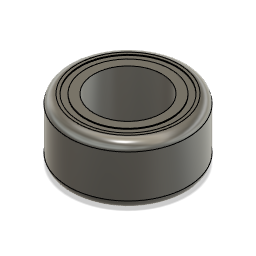
dualTriggerRemote v15 (Autodesk Fusion 360 archive; units mm, degrees)
design "smallBearing"
Autodesk Fusion 360 part; units mm, degrees
sketch "Sketch1" plane through (0, 0, 0) normal (0, 1, 0) x (1, 0, 0)
  circle A0 centre (0, 0) radius 7
  circle A1 centre (0, 0) radius 4
  dimension "d1" = 14
  dimension "d2" = 8
  constraint coincident A0.centre A1.centre
  measures "d1" diameter of A0
  measures "d2" diameter of A1
extrude "Extrude1" add sketch "Sketch1" along normal blind 7
fillet "Fillet1" radius 1 2 edges at (-6.5263, 0, 2.5313) (-6.5263, 7, 2.5313)
sketch "Sketch2" plane through (0, 7, 0) normal (0, 1, 0) x (-1, 0, 0)
  circle A0 centre (0, 0) radius 4
  circle A1 centre (0, 0) radius 6
  circle A2 centre (0, 0) radius 5.6638
  circle A3 centre (0, 0) radius 5
  constraint concentric A0 A2
  constraint concentric A0 A3
extrude "Extrude2" cut sketch "Sketch2" against normal blind 0.1 contours A2
sketch "Sketch3" plane through (0, 0, 0) normal (0, -1, 0) x (1, 0, 0)
  circle A0 centre (0, 0) radius 4
  circle A1 centre (0, 0) radius 6
  circle A2 centre (0, 0) radius 5
  circle A3 centre (0, 0) radius 5.6638
extrude "Extrude3" cut sketch "Sketch3" against normal blind 0.2 contours A3

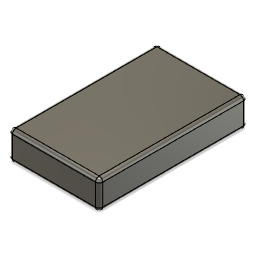
design "battery"
Autodesk Fusion 360 part; units mm, degrees
sketch "Sketch1" plane through (0, 0, 0) normal (0, 1, 0) x (1, 0, 0)
  line L0 (0, 0) -> (25, 0)
  line L1 (25, 0) -> (25, 41)
  line L2 (25, 41) -> (0, 41)
  line L3 (0, 41) -> (0, 0)
  dimension "d1" = 25
  dimension "d2" = 41
  constraint horizontal L0
  constraint vertical L1
  constraint horizontal L2
  constraint vertical L3
  constraint coincident L0.start L3.end
  measures "d1" distance of L0.start L0.end
  measures "d2" distance of L0.start L2.end
extrude "Extrude1" add sketch "Sketch1" along normal blind 8
fillet "Fillet1" radius 1 12 edges at (12.5, 8, 0) (25, 8, -20.5) (12.5, 8, -41) (0, 8, -20.5) (25, 0, -20.5) (25, 4, 0) (12.5, 0, 0) (0, 0, -20.5) (0, 4, 0) (0, 4, -41) (12.5, 0, -41) (25, 4, -41)
